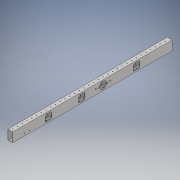
# Autodesk Inventor part: Drivetrain_length
Saved by Autodesk Inventor 2018 (Build 220112000, 112)
## iProperties
Created: 2018-09-05
Part Number: Drivetrain_length
Material: Generic
Document SubType Name: Modeling
Designer: baoan
Density: 1 g/cm^3
Appearance: Default
Author: baoan
Autodesk Inventor part; units mm, degrees
ref_plane "YZ Plane" through (0, 0, 0) normal (1, 0, 0) x (0, 1, 0)
ref_plane "XZ Plane" through (0, 0, 0) normal (0, 1, 0) x (-1, 0, 0)
ref_plane "XY Plane" through (0, 0, 0) normal (0, 0, 1) x (1, 0, 0)
sketch "Sketch1" plane through (0, 0, 0) normal (0, 0, 1) x (1, 0, 0)
  line L0 (-12.7, -25.4) -> (12.7, -25.4)
  line L1 (12.7, -25.4) -> (12.7, 25.4)
  line L2 (12.7, 25.4) -> (-12.7, 25.4)
  line L3 (-12.7, 25.4) -> (-12.7, -25.4)
  line L4 (-12.7, -25.4) -> (12.7, 25.4) construction
  line L5 (12.7, -25.4) -> (-12.7, 25.4) construction
  line L6 (-10.16, -22.86) -> (10.16, -22.86)
  line L7 (10.16, -22.86) -> (10.16, 22.86)
  line L8 (10.16, 22.86) -> (-10.16, 22.86)
  line L9 (-10.16, 22.86) -> (-10.16, -22.86)
  line L10 (-10.16, -22.86) -> (10.16, 22.86) construction
  line L11 (10.16, -22.86) -> (-10.16, 22.86) construction
  point P0 (0, 0)
  dimension "d0" = 25.4
  dimension "d1" = 50.8
  dimension "d2" = 20.32
  dimension "d3" = 45.72
  constraints: 24 end point, 4 midpoint, 4 parallel, 2 horizontal, 2 perpendicular
  measures "d0" distance of L2.end L1.end
  measures "d1" distance of L1.end L0.end
  measures "d2" distance of L8.end L7.end
  measures "d3" distance of L7.end L6.end
extrude "Extrusion1" add sketch "Sketch1" along normal mid plane 850.9
sketch "Sketch2" plane through (-12.7, 25.4, 425.45) normal (0, 1, 0) x (1, 0, 0)
  line L0 (25.4, 850.9) -> (25.4, 0) projected
  line L1 (25.4, 0) -> (0, 0) projected
  point P0 (12.7, 425.45)
  point P1 (12.7, 12.7)
  dimension "d6" = 12.7
  dimension "d7" = 12.7
  measures "d6" distance from line of L0 point (12.7, 12.7)
  measures "d7" distance from line of L1 point (12.7, 12.7)
hole "Hole1" at (0, 25.4, 412.75) direction (0, -1, 0) diameter 4.1402 end through all
pattern_linear "Rectangular Pattern1" count 36 spacing 25.4 along (0, 0, -1) of "Hole1"
sketch "Sketch4" plane through (12.7, -25.4, 425.45) normal (1, 0, 0) x (0, 0, -1)
  line L0 (850.9, 0) -> (0, 0) projected
  line L1 (850.9, 50.8) -> (850.9, 0) projected
  line L2 (0, 0) -> (0, 50.8) projected
  line L3 (179.3875, 7.9375) -> (201.6125, 7.9375)
  line L4 (207.9625, 14.2875) -> (207.9625, 36.5125)
  line L5 (201.6125, 42.8625) -> (179.3875, 42.8625)
  line L6 (173.0375, 36.5125) -> (173.0375, 14.2875)
  line L7 (173.0375, 7.9375) -> (207.9625, 42.8625) construction
  line L8 (207.9625, 7.9375) -> (173.0375, 42.8625) construction
  line L9 (357.1875, 7.9375) -> (379.4125, 7.9375)
  line L10 (385.7625, 14.2875) -> (385.7625, 36.5125)
  line L11 (379.4125, 42.8625) -> (357.1875, 42.8625)
  line L12 (350.8375, 36.5125) -> (350.8375, 14.2875)
  line L13 (350.8375, 7.9375) -> (385.7625, 42.8625) construction
  line L14 (385.7625, 7.9375) -> (350.8375, 42.8625) construction
  line L15 (649.2875, 7.9375) -> (671.5125, 7.9375)
  line L16 (677.8625, 14.2875) -> (677.8625, 36.5125)
  line L17 (671.5125, 42.8625) -> (649.2875, 42.8625)
  line L18 (642.9375, 36.5125) -> (642.9375, 14.2875)
  line L19 (642.9375, 7.9375) -> (677.8625, 42.8625) construction
  line L20 (677.8625, 7.9375) -> (642.9375, 42.8625) construction
  arc A0 (179.3875, 42.8625) -> (173.0375, 36.5125) centre (179.3875, 36.5125) ccw
  arc A1 (207.9625, 36.5125) -> (201.6125, 42.8625) centre (201.6125, 36.5125) ccw
  arc A2 (201.6125, 7.9375) -> (207.9625, 14.2875) centre (201.6125, 14.2875) ccw
  arc A3 (173.0375, 14.2875) -> (179.3875, 7.9375) centre (179.3875, 14.2875) ccw
  arc A4 (357.1875, 42.8625) -> (350.8375, 36.5125) centre (357.1875, 36.5125) ccw
  arc A5 (385.7625, 36.5125) -> (379.4125, 42.8625) centre (379.4125, 36.5125) ccw
  arc A6 (379.4125, 7.9375) -> (385.7625, 14.2875) centre (379.4125, 14.2875) ccw
  arc A7 (350.8375, 14.2875) -> (357.1875, 7.9375) centre (357.1875, 14.2875) ccw
  arc A8 (649.2875, 42.8625) -> (642.9375, 36.5125) centre (649.2875, 36.5125) ccw
  arc A9 (677.8625, 36.5125) -> (671.5125, 42.8625) centre (671.5125, 36.5125) ccw
  arc A10 (671.5125, 7.9375) -> (677.8625, 14.2875) centre (671.5125, 14.2875) ccw
  arc A11 (642.9375, 14.2875) -> (649.2875, 7.9375) centre (649.2875, 14.2875) ccw
  point P0 (425.45, 25.4)
  point P1 (482.6, 25.4)
  point P2 (506.4125, 25.4)
  point P3 (458.7875, 25.4)
  point P4 (190.5, 25.4)
  point P5 (368.3, 25.4)
  point P6 (660.4, 25.4)
  dimension "d27" = 25.4
  dimension "d28" = 368.3
  dimension "d36" = 23.8125
  dimension "d37" = 23.8125
  dimension "d45" = 190.5
  dimension "d46" = 177.8
  dimension "d47" = 190.5
  dimension "d48" = 34.925
  dimension "d49" = 34.925
  dimension "d50" = 34.925
  dimension "d51" = 34.925
  dimension "d52" = 34.925
  dimension "d53" = 34.925
  dimension "d54" = 6.35
  constraints: 36 end point, 24 point on circle, 24 point on line, 24 tangent, 12 centre point, 11 equal radius, 6 midpoint, 6 parallel, 5 horizontal alignment, 3 horizontal, 3 perpendicular
  measures "d27" distance from line of L0 point (482.6, 25.4)
  measures "d28" distance from line of L1 point (482.6, 25.4)
  measures "d36" distance of point (458.788, 25.4) point (482.6, 25.4)
  measures "d37" distance of point (506.413, 25.4) point (482.6, 25.4)
  measures "d45" distance from line of L2 point (190.5, 25.4)
  measures "d46" distance of point (368.3, 25.4) point (190.5, 25.4)
  measures "d47" distance from line of L1 point (660.4, 25.4)
  measures "d48" distance of L8.end L7.end
  measures "d49" distance of L7.end L8.start
  measures "d50" distance of L14.end L13.end
  measures "d51" distance of L13.end L14.start
  measures "d52" distance of L20.end L19.end
  measures "d53" distance of L19.end L20.start
  measures "d54" radius of A0
hole "Hole2" at (12.7, 0, -57.15) direction (-1, 0, 0) diameter 38.1 end through all
hole "Hole3" at (12.7, 0, -80.9625) at (12.7, 0, -33.3375) direction (-1, 0, 0) diameter 5.1054 end through all
extrude "Extrusion2" cut sketch "Sketch4" against normal through all
sketch "Sketch5" plane through (12.7, -25.4, 425.45) normal (1, 0, 0) x (0, 0, -1)
  line L0 (850.9, 0) -> (0, 0) projected
  circle A0 centre (458.7875, 25.4) radius 2.5527 projected
  circle A1 centre (506.4125, 25.4) radius 2.5527 projected
  line L1 (850.9, 50.8) -> (0, 50.8) projected
  point P0 (425.45, 25.4)
  point P1 (444.3962, 27.1938)
  point P2 (520.8038, 27.1938)
  dimension "d58" = 14.3913
  dimension "d60" = 14.3913
  dimension "d61" = 23.6062
  dimension "d62" = 23.6062
  measures "d58" horizontal distance of A0.centre point (444.396, 27.194)
  measures "d60" horizontal distance of A1.centre point (520.804, 27.194)
  measures "d61" distance from line of L1 point (520.804, 27.194)
  measures "d62" distance from line of L1 point (444.396, 27.194)
hole "Hole4" at (12.7, 1.7938, -18.9462) at (12.7, 1.7938, -95.3538) direction (-1, 0, 0) diameter 6.604 end through all
sketch "Sketch6" plane through (-12.7, -25.4, 425.45) normal (-1, 0, 0) x (0, 0, 1)
  line L0 (-101.6, -25.4) -> (-101.6, 25.4)
  line L1 (-101.6, 25.4) -> (76.2, 25.4)
  point P0 (-425.45, 25.4)
  point P1 (-63.5, 12.7)
  point P2 (-88.9, 12.7)
  dimension "d70" = 25.4
  dimension "d71" = 12.7
  dimension "d72" = 12.7
  constraints: 4 end point, 1 horizontal, 1 vertical, 3 other
  measures "d70" distance of point (-63.5, 12.7) point (-88.9, 12.7)
  measures "d71" distance from line of L0 point (-88.9, 12.7)
  measures "d72" distance from line of L1 point (-88.9, 12.7)
hole "Hole5" at (-12.7, -12.7, 361.95) at (-12.7, -12.7, 336.55) direction (1, 0, 0) diameter 4.1402 end through all
equation "\"d60\" = d58"
equation "\"d62\" = d61"
body "Solid1"
